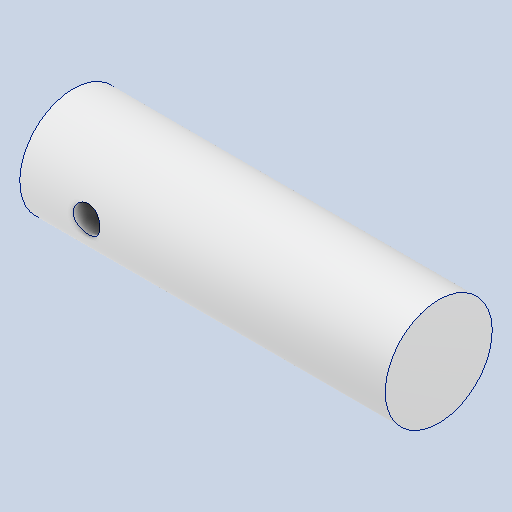
# Autodesk Inventor part: roller-hand-v2-Shaft-m
Saved by Autodesk Inventor 2025.1 (Build 291241000, 241)
## iProperties
Created: 2024-10-06
Part Number: roller-hand-v2-Shaft-m
Material: アルミニウム 6061
Document SubType Name: Modeling
Designer: haruy
Density: 2.7 g/cm^3
Appearance: アルミニウム - フラット
Author: haruy
Autodesk Inventor part; units mm, degrees
ref_plane "YZ Plane" through (0, 0, 0) normal (1, 0, 0) x (0, 1, 0)
ref_plane "XZ Plane" through (0, 0, 0) normal (0, 1, 0) x (-1, 0, 0)
sketch "スケッチ1" plane through (0, 0, 0) normal (1, 0, 0) x (0, 1, 0)
  circle A0 centre (0, 0) radius 6
  dimension "d0" = 12
  constraints: 1 centre point, 1 coincident
  measures "d0" diameter of A0
extrude "押し出し1" add sketch "スケッチ1" along normal blind 41
ref_plane "作業平面1" through (0, 0, 6) normal (0, 0, 1) x (1, 0, 0)
sketch "スケッチ2" plane through (0, 0, 6) normal (0, 0, 1) x (1, 0, 0)
  line L0 (0, -6) -> (0, 6) projected
  point P0 (0, 0)
  point P1 (7.5, 0)
  dimension "d3" = 7.5
  measures "d3" distance from line of point (7.5, 0) L0
hole "穴1" at (7.5, 0, 6) direction (0, 0, -1) diameter 3 end through all
